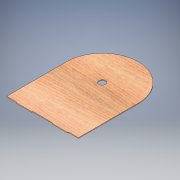
# Autodesk Inventor part: turretSidePlateOne
Saved by Autodesk Inventor 2018 (Build 220112000, 112)
## iProperties
Created: 2019-02-27
Part Number: turretSidePlateOne
Material: Generic
Document SubType Name: Modeling
Designer: snipe
Density: 1 g/cm^3
Appearance: Default
Author: snipe
Autodesk Inventor part; units mm, degrees
ref_plane "YZ Plane" through (0, 0, 0) normal (1, 0, 0) x (0, 1, 0)
ref_plane "XZ Plane" through (0, 0, 0) normal (0, 1, 0) x (-1, 0, 0)
ref_plane "XY Plane" through (0, 0, 0) normal (0, 0, 1) x (1, 0, 0)
sketch "Sketch1" plane through (0, 0, 0) normal (0, 1, 0) x (-1, 0, 0)
  line L0 (0, -234.315) -> (0, 339.09) projected
  line L1 (-213.36, 0) -> (213.36, 0) projected
  line L2 (213.36, 0) -> (-213.36, 0) projected
  line L3 (0, -234.315) -> (0, 339.09) projected
  line L4 (152.4, 254) -> (-152.4, 254)
  line L5 (-152.4, 254) -> (-152.4, 0)
  line L6 (152.4, 0) -> (152.4, 254)
  arc A0 (-152.4, 0) -> (152.4, 0) centre (0, 0) ccw
  line L7 (107.95, 254) -> (44.45, 254) construction
  line L8 (107.95, 257.175) -> (44.45, 257.175)
  line L9 (44.45, 250.825) -> (107.95, 250.825)
  arc A1 (107.95, 250.825) -> (107.95, 257.175) centre (107.95, 254) ccw
  arc A2 (44.45, 257.175) -> (44.45, 250.825) centre (44.45, 254) ccw
  line L10 (-44.45, 254) -> (-107.95, 254) construction
  line L11 (-44.45, 257.175) -> (-107.95, 257.175)
  line L12 (-107.95, 250.825) -> (-44.45, 250.825)
  arc A3 (-44.45, 250.825) -> (-44.45, 257.175) centre (-44.45, 254) ccw
  arc A4 (-107.95, 257.175) -> (-107.95, 250.825) centre (-107.95, 254) ccw
  circle A5 centre (0, 0) radius 14.2875
  point P0 (76.2, 254)
  point P1 (-76.2, 254)
  point P2 (0, -152.4)
  dimension "d2" = 63.5
  dimension "d3" = 6.35
  dimension "d4" = 63.5
  dimension "d5" = 6.35
  dimension "d7" = 76.2
  dimension "d8" = 304.8
  dimension "d9" = 76.2
  dimension "d10" = 28.575
  dimension "d11" = 406.4
  constraints: 22 end point, 11 point on circle, 10 tangent, 6 centre point, 4 point on line, 3 parallel, 2 coincident, 2 midpoint, 1 horizontal, 1 perpendicular
  measures "d2" distance of L7.start L7.end
  measures "d3" diameter of A2
  measures "d4" distance of L10.start L10.end
  measures "d5" diameter of A4
  measures "d7" distance from line of L0 point (76.2, 254)
  measures "d8" distance of L4.start L4.end
  measures "d9" distance from line of point (-76.2, 254) L0
  measures "d10" diameter of A5
  measures "d11" distance from line of L4 point (0, -152.4)
extrude "Extrusion1" add sketch "Sketch1" along normal blind 3.175 contours A0 L1 A5 L0 | L0 A5 L1 A0 | L5 L4 A4 L12 A3 L0 A5 L1 | L1 A5 L0 L4 A2 L9 A1 L6 | A4 L11 A3 L4 | L4 A3 L12 A4 | A1 L9 A2 L4 | L4 A2 L8 A1
body "Solid1"
